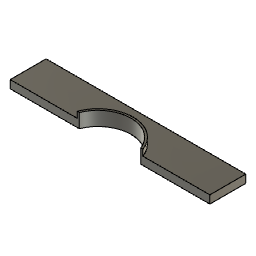
DISP_Ring_support v1 (Autodesk Fusion 360 design; units mm, degrees)
Autodesk Fusion 360 part; units mm, degrees
sketch "Sketch1" plane through (0, 0, 0) normal (0, 0, 1) x (1, 0, 0)
  circle A0 centre (0, 0) radius 16.5
  circle A1 centre (0, 0) radius 12.5
  dimension "d1" = 33
  dimension "d2" = 25
  constraint coincident A0.centre A1.centre
  measures "d1" diameter of A0
  measures "d2" diameter of A1
extrude "Extrude1" add sketch "Sketch1" along normal blind 8 makes body 1
extrude "Extrude2" cut 1 faces at (15.1052, -0.8197, 8) along direction (0, 0, -1) blind 37 on bodies 1 bodies 1
sketch "Sketch2" plane through (0, 0, 0) normal (0, 0, 1) x (1, 0, 0)
  circle A0 centre (0, 0) radius 17.5
  circle A1 centre (0, 0) radius 21
  line L0 (0, 0) -> (-21, 0)
  line L1 (0, 0) -> (21, 0)
  circle A2 centre (0, 0) radius 21 construction
  circle A3 centre (0, 21) radius 7.5 construction
  line L2 (0, 21) -> (0, 6) construction
  line L3 (0, 6) -> (20.1246, 6) construction
  line L4 (0, 6) -> (-20.1246, 6) construction
  line L5 (0, 6) -> (50, 6)
  line L6 (0, 6) -> (-15, 6)
  line L7 (0, 6) -> (-50, 6)
  circle A4 centre (0, 6) radius 9 construction
  line L8 (0, 6) -> (0, 24) construction
  line L9 (0, 24) -> (-50, 24)
  line L10 (-50, 24) -> (-50, 6)
  line L11 (0, 24) -> (50, 24)
  line L12 (50, 24) -> (50, 6)
  dimension "d7" = 35
  dimension "d8" = 42
  dimension "d9" = 15
  dimension "d10" = 15
  dimension "d11" = 50
  dimension "d12" = 15
  dimension "d13" = 50
  dimension "d14" = 18
  dimension "d15" = 18
  constraint coincident A0.centre A1.centre
  constraint concentric A0 A1
  constraint coincident A1 L0.end
  constraint horizontal L0
  constraint coincident A1 L1.end
  constraint parallel L0 L1
  constraint coincident A1 A3.centre
  constraint coincident A3.centre L2.start
  constraint vertical L2
  constraint coincident A2 L3.end
  constraint perpendicular L2 L3
  constraint coincident A1 L4.end
  constraint perpendicular L2 L4
  constraint perpendicular L2 L5
  constraint perpendicular L2 L6
  constraint perpendicular L2 L7
  constraint coincident L2.end L3.start
  constraint parallel L2 L8
  constraint perpendicular L8 L9
  constraint perpendicular L8 L11
  measures "d7" diameter of A0
  measures "d8" diameter of A1
  measures "d9" diameter of A3
  measures "d10" distance of A3.centre L2.end
  measures "d11" distance of L2.end L5.end
  measures "d12" distance of L2.end L6.end
  measures "d13" distance of L2.end L7.end
  measures "d14" diameter of A4
  measures "d15" distance of L2.end L8.end
extrude "Extrude3" add sketch "Sketch2" against normal blind 4 contours A0 A1 L5 L7 | A1 L5 L7 L9 L10 L11 L12 bodies 1
sketch "Sketch3" plane through (0, 0, 0) normal (0, 0, 1) x (-1, 0, 0)
  line L0 (-50, -24) -> (50, -24)
  line L1 (50, -24) -> (50, -6)
  line L2 (50, -6) -> (16.4393, -6)
  arc A0 (-16.4393, -6) -> (16.4393, -6) centre (0, 0) ccw
  line L3 (-16.4393, -6) -> (-50, -6)
  line L4 (-50, -6) -> (-50, -24)
  circle A1 centre (0, 0) radius 16.5
  circle A2 centre (0, 0) radius 17.5
  line L5 (16.4393, -6) -> (-16.4393, -6)
  dimension "d18" = 33
  constraint concentric A0 A1
  constraint concentric A1 A2
  constraint coincident L2.end A0.end
  constraint coincident A0.start L3.start
  measures "d18" diameter of A1
extrude "Extrude4" add sketch "Sketch3" along normal blind 3 separate body contours A0 A1 A2 L5 makes body 2
extrude "Extrude5" add 1 faces at (-1.2395, 16.7567, 0) along direction (0, 0, -1) blind 2 on bodies 2 bodies 2 1
extrude "Extrude6" add 1 faces at (-1.2395, 16.7567, -2) along direction (0, 0, -1) blind 2 on bodies 2 bodies 2
